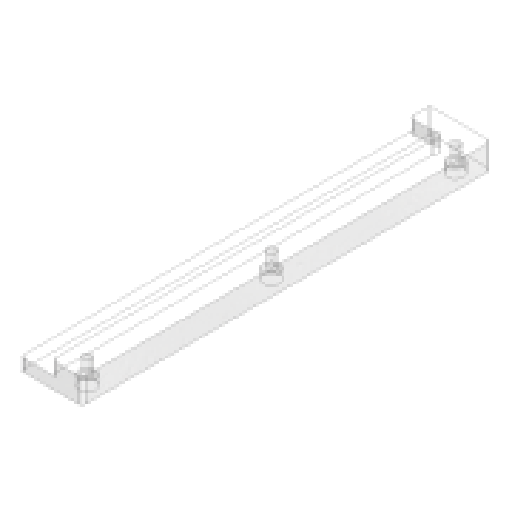
# Autodesk Inventor part: DLT-01-234
Saved by Autodesk Inventor 2025.2 (Build 292293000, 293)
## iProperties
Company: Delta
Created: 2024-11-01
Part Number: DLT-01-234
Material: Acrílico TP
Document SubType Name: Modeling
Designer: Willian Pinheiro
Density: 1.19 g/cm^3
Appearance: Transparent - Clear
Project: DLT-01
Description: Guia Pressor R
Mass: 56.1859 g
Surface Area: 159.718 cm^2
Volume: 47.2151 cm^3
Acabamento: N/A
Dimensões: 10 x 25 x 200 mm
Total: 1
Author: Willian Pinheiro
Revision Number: 00
Autodesk Inventor part; units mm, degrees
ref_plane "YZ Plane" through (0, 0, 0) normal (1, 0, 0) x (0, 1, 0)
ref_plane "XZ Plane" through (0, 0, 0) normal (0, 1, 0) x (-1, 0, 0)
ref_plane "XY Plane" through (0, 0, 0) normal (0, 0, 1) x (1, 0, 0)
sketch "Sketch1" plane through (0, 0, 0) normal (0, 0, 1) x (1, 0, 0)
  line L0 (-21, 0) -> (21, 0) construction
  line L1 (0, -140) -> (0, 140) construction
  line L2 (-15, 100) -> (15, 100)
  line L3 (15, 100) -> (15, -100)
  line L4 (15, -100) -> (-15, -100)
  line L5 (-15, -100) -> (-15, 100)
  line L6 (-0.1, 90.05) -> (15, 90.05)
  line L7 (15, 90.05) -> (15, -100)
  line L8 (15, -100) -> (-0.1, -100)
  line L9 (-0.1, -100) -> (-0.1, 90.05)
  circle A0 centre (1.9, 88.05) radius 3
  line L10 (9.9, 100) -> (9.9, 90.05)
  point P0 (0, 0)
  point P1 (15, 90.05)
  point P2 (4.1361, 90.05)
  point P3 (-0.1, 85.8139)
  dimension "d0" = 30
  dimension "d1" = 200
  dimension "d2" = 9.95
  dimension "d3" = 15.1
  dimension "d16" = 2
  dimension "d17" = 6
  dimension "d18" = 2
  dimension "d23" = 14.9
  dimension "d26" = 10
  constraints: 18 end point, 4 parallel, 3 perpendicular, 2 horizontal, 2 point on line, 1 centre point, 2 other
  measures "d0" distance between parallel lines of L5 L3
  measures "d1" distance of L4.end L2.start
  measures "d2" distance between parallel lines of L2 L6
  measures "d3" distance between parallel lines of L3 L9
  measures "d16" distance from line of L9 A0.centre
  measures "d17" diameter of A0
  measures "d18" distance from line of A0.centre L6
  measures "d23" distance between parallel lines of L5 L9
  measures "d26" distance between parallel lines of L9 L10
extrude "Extrusion1" add sketch "Sketch1" against normal blind 10
extrude "Extrusion2" cut sketch "Sketch1" against normal blind 6.1 contours L2 L3 L6 L10 | L6 L3 L4 L9 A0 | A0 L9 L6 | L6 L9 A0
sketch "Sketch2" plane through (0, 0, -10) normal (0, 0, -1) x (-1, 0, 0)
  line L0 (-4.1361, 90.05) -> (-9.9, 90.05) construction
  line L1 (-9.9, 100) -> (15, 100) construction
  line L2 (15, 100) -> (15, -100) construction
  line L3 (15, -100) -> (0.1, -100) construction
  line L4 (0.1, -100) -> (0.1, 85.8139) construction
  line L5 (7.5, -100) -> (7.5, 100) construction
  line L6 (21, 0) -> (-21, 0) construction
  arc A0 (0.1, 85.8139) -> (-4.1361, 90.05) centre (-1.9, 88.05) ccw projected
  line L7 (-9.9, 90.05) -> (-9.9, 100) projected
  point P0 (0, 0)
  point P1 (7.5, -90)
  point P2 (7.5, 90)
  point P3 (7.5, 0)
  dimension "d8" = 180
  dimension "d24" = 7.5
  constraints: 2 end point, 2 point on line, 1 midpoint, 1 perpendicular, 1 symmetric about line
  measures "d8" distance of point (7.5, 90) point (7.5, -90)
  measures "d24" distance between parallel lines of L5 L2
hole "Hole1" at (-7.5, -90, -10) at (-7.5, 0, -10) at (-7.5, 90, -10) direction (0, 0, 1) diameter 4.5 end through all counterbore diameter 8 counterbore depth 4.6 clearance for "Socket Head Cap Screw ISO 4762" size "M4" standard "ISO"
mirror "Mirror1" about plane through (0, 0, 0) normal (1, 0, 0) remove original yes
fillet "Fillet1" radius 2 6 edges at (15, -100, -5) (15, 100, -5) (0.1, -100, -3.05) (-4.1361, 90.05, -3.05) (0.1, 85.8139, -3.05) (-9.9, 90.05, -3.05)
fillet "Fillet1" radius 1 3 edges at (-15, 100, -8.05) (-15, -100, -8.05) (-9.9, 100, -3.05)
equation "\"d16\" = 0.333333 * d17"
equation "\"d18\" = d16"
body "Solid1"
